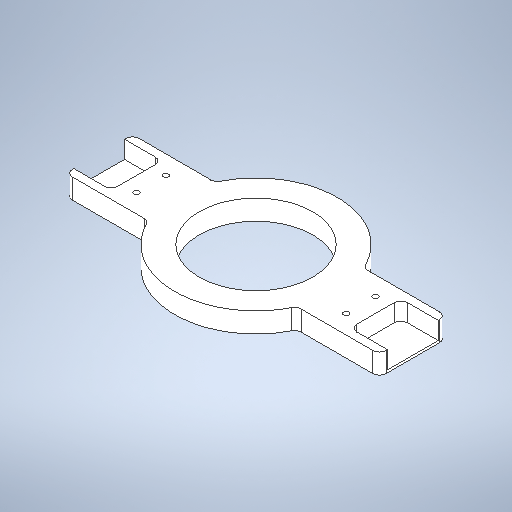
# Autodesk Inventor part: Plastic Head Thing Bottom
Saved by Autodesk Inventor 2025 (Build 290162000, 162)
## iProperties
Created: 2025-06-24
Part Number: Plastic Head Thing Bottom
Material: Generic
Document SubType Name: Modeling
Designer: mumin
Density: 1 g/cm^3
Appearance: Default
Author: mumin
Autodesk Inventor part; units mm, degrees
ref_plane "YZ Plane" through (0, 0, 0) normal (1, 0, 0) x (0, 1, 0)
ref_plane "XZ Plane" through (0, 0, 0) normal (0, 1, 0) x (-1, 0, 0)
ref_plane "XY Plane" through (0, 0, 0) normal (0, 0, 1) x (1, 0, 0)
sketch "Sketch1" plane through (0, 0, 0) normal (0, 1, 0) x (-1, 0, 0)
  circle A0 centre (0, 0) radius 42.5
  arc A1 (55.6417, 25) -> (-55.6417, 25) centre (0, 0) ccw
  line L0 (0, 0) -> (0, -61)
  line L1 (0, 0) -> (0, 0)
  line L2 (-117.5, 25) -> (-117.5, -25)
  line L3 (117.5, -25) -> (117.5, 25)
  line L4 (117.5, 25) -> (-117.5, -25) construction
  line L5 (-117.5, 25) -> (117.5, -25) construction
  line L6 (117.5, 25) -> (55.6417, 25)
  line L7 (-55.6417, 25) -> (-117.5, 25)
  line L8 (55.6417, -25) -> (117.5, -25)
  line L9 (-117.5, -25) -> (-55.6417, -25)
  arc A2 (-55.6417, -25) -> (55.6417, -25) centre (0, 0) ccw
  point P0 (0, -61)
  dimension "d0" = 85
  dimension "d1" = 61
  dimension "d2" = 235
  dimension "d3" = 50
  constraints: 20 end point, 5 coincident, 5 parallel, 4 point on circle, 3 centre point, 3 horizontal, 2 midpoint, 2 perpendicular, 1 vertical, 1 vertical alignment
  measures "d0" diameter of A0
  measures "d1" radius of A1
  measures "d2" distance of L5.end L2.end
  measures "d3" distance of L2.end L2.start
extrude "Extrusion1" add sketch "Sketch1" along normal blind 15
sketch "Sketch2" plane through (0, 15, 0) normal (0, 1, 0) x (1, 0, 0)
  line L0 (-117.5, 25) -> (-117.5, -25) projected
  line L1 (-117.5, 19) -> (-94.5, 19)
  line L2 (-89.5, 14) -> (-89.5, -14)
  line L3 (-94.5, -19) -> (-117.5, -19)
  arc A0 (-89.5, 14) -> (-94.5, 19) centre (-94.5, 14) ccw
  arc A1 (-94.5, -19) -> (-89.5, -14) centre (-94.5, -14) ccw
  line L4 (-117.5, 25) -> (-117.5, -25) projected
  line L5 (-164.5, 0) -> (164.5, 0) projected
  point P0 (0, 0)
  dimension "d6" = 5
  dimension "d7" = 38
  dimension "d8" = 28
  constraints: 6 end point, 4 point on circle, 4 tangent, 2 centre point, 2 perpendicular, 2 point on line, 1 equal radius, 1 horizontal, 1 other
  measures "d6" radius of A0
  measures "d7" distance between parallel lines of L3 L1
  measures "d8" distance between parallel lines of L2 L0
extrude "Extrusion2" cut sketch "Sketch2" against normal blind 13.1
mirror "Mirror1" about plane through (0, 0, 0) normal (1, 0, 0) of "Extrusion2"
sketch "Sketch3" plane through (0, 0, 0) normal (0, -1, 0) x (1, 0, 0)
  line L0 (-117.5, -25) -> (-117.5, 25) projected
  line L1 (-164.5, 0) -> (164.5, 0) projected
  point P0 (0, 0)
  point P1 (-78.5, -11)
  point P2 (-78.5, 11)
  dimension "d19" = 39
  dimension "d22" = 11
  constraints: 1 symmetric about line
  measures "d19" distance from line of L0 point (-78.5, -11)
  measures "d22" distance from line of L1 point (-78.5, -11)
hole "Hole1" at (-78.5, 0, -11) at (-78.5, 0, 11) direction (0, 1, 0) diameter 4 depth 15 counterbore diameter 8 counterbore depth 6
mirror "Mirror2" about plane through (0, 0, 0) normal (1, 0, 0) of "Hole1"
fillet "Fillet1" radius 5 8 edges at (117.5, 7.5, -25) (117.5, 7.5, 25) (55.6417, 7.5, -25) (-55.6417, 7.5, -25) (-117.5, 7.5, -25) (55.6417, 7.5, 25) (-55.6417, 7.5, 25) (-117.5, 7.5, 25)
ref_plane "Work Plane1" through (0, 0, 0) normal (1, 0, 0) x (0, 1, 0)
body "Solid1"
